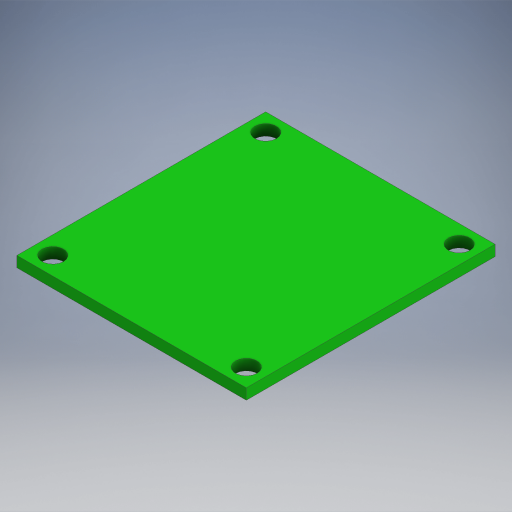
# Autodesk Inventor part: Плата драйвера
Saved by Autodesk Inventor 2023 (Build 270158000, 158)
## iProperties
Created: 2023-01-19
Part Number: Плата драйвера
Material: Типовые
Document SubType Name: Modeling
Designer: Admin
Density: 1 g/cm^3
Appearance: По умолчанию
Author: Admin
Autodesk Inventor part; units mm, degrees
ref_plane "YZ Plane" through (0, 0, 0) normal (1, 0, 0) x (0, 1, 0)
ref_plane "XZ Plane" through (0, 0, 0) normal (0, 1, 0) x (-1, 0, 0)
ref_plane "XY Plane" through (0, 0, 0) normal (0, 0, 1) x (1, 0, 0)
sketch "Эскиз1" plane through (0, 0, 0) normal (0, 1, 0) x (-1, 0, 0)
  line L0 (-16, 17.35) -> (16, 17.35)
  line L1 (16, 17.35) -> (16, -17.35)
  line L2 (16, -17.35) -> (-16, -17.35)
  line L3 (-16, -17.35) -> (-16, 17.35)
  line L4 (-16, 17.35) -> (16, -17.35) construction
  line L5 (16, 17.35) -> (-16, -17.35) construction
  circle A0 centre (13.5, 14.85) radius 1.5
  circle A1 centre (13.5, -14.85) radius 1.5
  circle A2 centre (-13.5, -14.85) radius 1.5
  circle A3 centre (-13.5, 14.85) radius 1.5
  point P0 (0, 0)
  dimension "d0" = 34.7
  dimension "d1" = 32
  dimension "d2" = 3
  dimension "d3" = 1
  dimension "d4" = 1
  dimension "d5" = 1
  dimension "d6" = 1
  constraints: 12 end point, 4 centre point, 3 equal radius, 2 horizontal alignment, 2 midpoint, 2 parallel, 2 vertical alignment, 1 horizontal, 1 perpendicular
  measures "d0" distance of L0.end L1.end
  measures "d1" distance of L1.end L2.end
  measures "d2" diameter of A1
  measures "d3" distance edge to line of A1 L1
  measures "d4" distance edge to line of A1 L2
  measures "d5" distance edge to line of A2 L3
  measures "d6" distance edge to line of A3 L0
extrude "Выдавливание1" add sketch "Эскиз1" along normal blind 1.5
